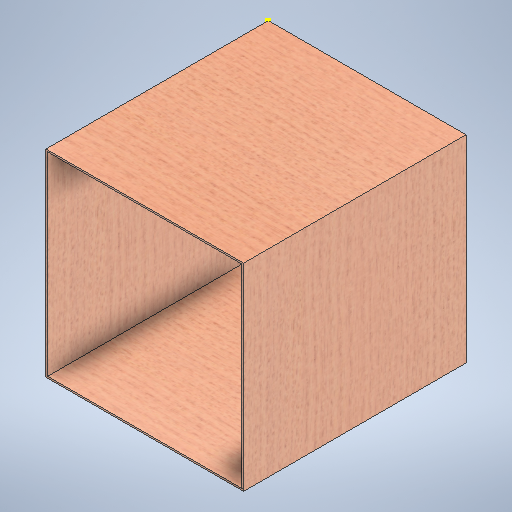
# Autodesk Inventor part: Caja grande
Saved by Autodesk Inventor 2025.1 (Build 291241000, 241)
## iProperties
Created: 2025-02-26
Part Number: Caja grande
Material: Generic
Document SubType Name: Modeling
Designer: yovan
Density: 1 g/cm^3
Appearance: Default
Author: yovan
Autodesk Inventor part; units mm, degrees
ref_plane "YZ Plane" through (0, 0, 0) normal (1, 0, 0) x (0, 1, 0)
ref_plane "XZ Plane" through (0, 0, 0) normal (0, 1, 0) x (-1, 0, 0)
ref_plane "XY Plane" through (0, 0, 0) normal (0, 0, 1) x (1, 0, 0)
sketch "Sketch1" plane through (0, 0, 0) normal (1, 0, 0) x (0, 1, 0)
  line L0 (0, 0) -> (240, 0)
  line L1 (240, 0) -> (240, 270)
  line L2 (240, 270) -> (0, 270)
  line L3 (0, 270) -> (0, 0)
  dimension "d0" = 240
  dimension "d1" = 270
  constraints: 8 end point, 2 parallel, 1 horizontal, 1 perpendicular
  measures "d0" distance of L2.end L1.end
  measures "d1" distance of L1.end L0.end
extrude "Extrusion1" add sketch "Sketch1" along normal blind 240
shell "Shell1" thickness 2 removed faces 1 at (80, 160, 270)
sketch "Sketch2" plane through (0, 240, 270) normal (0, 1, 0) x (1, 0, 0)
  point P0 (0, 270)
body "Solid1"
